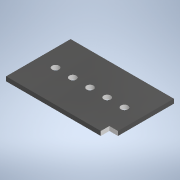
# Autodesk Inventor part: sheild
Saved by Autodesk Inventor 2021 (Build 250183000, 183)
## iProperties
Created: 2021-01-28
Part Number: sheild
Material: Generic
Document SubType Name: Modeling
Designer: Ryan
Density: 1 g/cm^3
Appearance: Default
Author: Ryan
Autodesk Inventor part; units mm, degrees
ref_plane "YZ Plane" through (0, 0, 0) normal (1, 0, 0) x (0, 1, 0)
ref_plane "XZ Plane" through (0, 0, 0) normal (0, 1, 0) x (-1, 0, 0)
ref_plane "XY Plane" through (0, 0, 0) normal (0, 0, 1) x (1, 0, 0)
sketch "Sketch1" plane through (0, 0, 0) normal (0, 1, 0) x (-1, 0, 0)
  line L0 (38.1, 23.7998) -> (-38.1, 23.7998)
  line L1 (-38.1, 23.7998) -> (-38.1, -23.7998)
  line L2 (-38.1, -23.7998) -> (38.1, -23.7998)
  line L3 (38.1, -23.7998) -> (38.1, 23.7998)
  point P0 (0, 0)
  dimension "d0" = 23.7998
  dimension "d1" = 47.5996
  dimension "d2" = 76.2
  dimension "d3" = 38.1
  constraints: 8 end point, 2 parallel, 1 horizontal, 1 perpendicular
  measures "d0" distance from line of point (0, 0) L2
  measures "d1" distance of L2.end L0.start
  measures "d2" distance of L1.end L2.end
  measures "d3" distance from line of L3 point (0, 0)
extrude "Extrusion1" add sketch "Sketch1" along normal blind 3.175
sketch "Sketch3" plane through (0, 3.175, 0) normal (0, 1, 0) x (1, 0, 0)
  line L0 (-38.1, 23.7998) -> (-38.1, -23.7998) projected
  line L1 (-38.1, 0) -> (-25.4, 0) construction
  line L2 (-25.4, 0) -> (-12.7, 0) construction
  line L3 (-12.7, 0) -> (0, 0) construction
  line L4 (0, 0) -> (12.7, 0) construction
  line L5 (12.7, 0) -> (25.4, 0) construction
  line L6 (25.4, 0) -> (38.1, 0) construction
  line L7 (38.1, -23.7998) -> (38.1, 23.7998) projected
  circle A0 centre (-25.4, 0) radius 1.905
  circle A1 centre (-12.7, 0) radius 1.905
  circle A2 centre (0, 0) radius 1.905
  circle A3 centre (12.7, 0) radius 1.905
  circle A4 centre (25.4, 0) radius 1.905
  point P0 (0, 0)
  dimension "d13" = 12.7
  dimension "d14" = 3.81
  constraints: 12 end point, 5 centre point, 5 coincident, 4 collinear, 4 equal radius, 4 point on line, 2 midpoint, 1 horizontal
  measures "d13" distance of L1.end L2.end
  measures "d14" diameter of A0
extrude "Extrusion3" cut sketch "Sketch3" against normal blind 25.4
sketch "Sketch4" plane through (0, 3.175, 0) normal (0, 1, 0) x (1, 0, 0)
  line L0 (-38.1, -23.7998) -> (38.1, -23.7998) projected
  line L1 (38.1, -23.7998) -> (31.75, -23.7998)
  line L2 (31.75, -23.7998) -> (31.75, -17.4498)
  line L3 (31.75, -17.4498) -> (38.1, -17.4498)
  line L4 (38.1, -17.4498) -> (38.1, -23.7998)
  point P0 (0, 0)
  dimension "d17" = 6.35
  constraints: 8 end point, 2 parallel, 2 perpendicular, 1 horizontal
  measures "d17" distance of L2.end L3.end
extrude "Extrusion4" cut sketch "Sketch4" against normal blind 25.4
equation "\"d0\" = 0.5 * d1"
equation "\"d3\" = 0.5 * d2"
body "Solid1"
